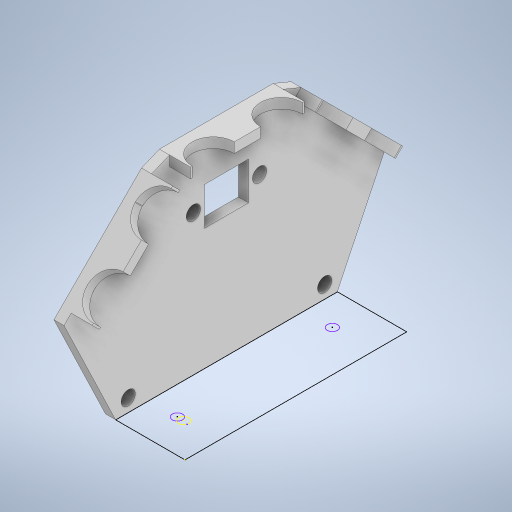
# Autodesk Inventor part: Top front deck
Saved by Autodesk Inventor 2024 (Build 280153000, 153)
## iProperties
Created: 2025-05-10
Part Number: Top front deck
Material: Generic
Document SubType Name: Modeling
Designer: arikm
Density: 1 g/cm^3
Appearance: Default
Author: arikm
Autodesk Inventor part; units mm, degrees
ref_plane "YZ Plane" through (0, 0, 0) normal (1, 0, 0) x (0, 1, 0)
ref_plane "XZ Plane" through (0, 0, 0) normal (0, 1, 0) x (-1, 0, 0)
ref_plane "XY Plane" through (0, 0, 0) normal (0, 0, 1) x (1, 0, 0)
sketch "Sketch1" plane through (0, 0, 0) normal (0, 1, 0) x (-1, 0, 0)
  line L0 (0, 0) -> (27.4, 0)
  line L1 (27.4, 0) -> (27.4, -87.7)
  line L2 (27.4, -87.7) -> (0, -87.7)
  line L3 (0, -87.7) -> (0, 0)
  line L4 (13.7, 0) -> (13.7, -13.2)
  line L5 (13.7, -87.7) -> (13.7, -74.5)
  circle A0 centre (13.7, -13.2) radius 2
  circle A1 centre (13.7, -74.5) radius 2
  dimension "d0" = 27.4
  dimension "d1" = 87.7
  dimension "d2" = 13.2
  dimension "d4" = 4
  dimension "d6" = 4
  constraints: 12 end point, 2 centre point, 2 coincident, 2 midpoint, 2 parallel, 2 vertical, 1 horizontal, 1 perpendicular
  measures "d0" distance of L1.end L2.end
  measures "d1" distance of L0.end L1.end
  measures "d2" distance of L4.start L4.end
  measures "d4" diameter of A0
  measures "d6" diameter of A1
extrude "Extrusion1" add sketch "Sketch1" along normal blind 10
sketch "Sketch2" plane through (0, 0, 0) normal (0, -1, 0) x (1, 0, 0)
  circle A0 centre (-13.7, -13.2) radius 2 projected
  circle A1 centre (-13.7, -13.2) radius 4.5
  circle A2 centre (-13.7, -74.5) radius 2 projected
  circle A3 centre (-13.7, -74.5) radius 4.5
  point P0 (0, 0)
  dimension "d9" = 9
  dimension "d10" = 9
  constraints: 2 centre point, 2 coincident
  measures "d9" diameter of A1
  measures "d10" diameter of A3
extrude "Extrusion2" cut sketch "Sketch2" against normal blind 3
sketch "Sketch3" plane through (0, 10, 0) normal (0, 1, 0) x (1, 0, 0)
  line L0 (0, 0) -> (0, 87.7) projected
  line L1 (0, 87.7) -> (-27.4, 87.7) projected
  line L2 (0, 0) -> (-27.4, 0)
  line L3 (-27.4, 0) -> (-27.4, 87.7)
  line L4 (-27.4, 87.7) -> (0, 87.7)
  line L5 (0, 87.7) -> (0, 0)
  circle A0 centre (-11.7, 12.5929) radius 0.0901
  circle A1 centre (-13.7, 13.2) radius 2 projected
  constraints: 8 end point, 2 parallel, 1 centre point, 1 horizontal, 1 perpendicular, 1 tangent
sketch "Sketch4" plane through (0, 0, 0) normal (0, -1, 0) x (1, 0, 0)
  line L0 (-27.4, -87.7) -> (-27.4, 0) projected
  line L1 (-27.4, -43.85) -> (0, -43.85)
  line L2 (0, 0) -> (0, -87.7) projected
  circle A0 centre (-13.7, -13.2) radius 2 projected
  line L3 (-13.7, -13.2) -> (-13.7, -26.4)
  line L4 (-13.7, -26.4) -> (0, -26.4)
  line L5 (0, -26.4) -> (0, -43.85)
  line L6 (0, -43.85) -> (-13.7, -43.85)
  line L7 (-13.7, -43.85) -> (-13.7, -26.4)
  line L8 (-13.7, -26.4) -> (-27.4, -26.4)
  line L9 (-27.4, -26.4) -> (-27.4, -43.85)
  line L10 (-27.4, -43.85) -> (-13.7, -43.85)
  line L11 (-13.7, -43.85) -> (-13.7, -26.4)
  circle A1 centre (-13.7, -74.5) radius 2 projected
  line L12 (-13.7, -74.5) -> (-13.7, -61.3)
  line L13 (-13.7, -43.85) -> (-13.7, -61.3)
  line L14 (-13.7, -61.3) -> (0, -61.3)
  line L15 (0, -61.3) -> (0, -43.85)
  line L16 (0, -43.85) -> (-13.7, -43.85)
  line L17 (-13.7, -43.85) -> (-13.7, -61.3)
  line L18 (-13.7, -43.85) -> (-27.4, -43.85)
  line L19 (-27.4, -43.85) -> (-27.4, -61.3)
  line L20 (-27.4, -61.3) -> (-13.7, -61.3)
  line L21 (-13.7, -61.3) -> (-13.7, -43.85)
  line L22 (0, -26.4) -> (-27.4, -26.4)
  line L23 (-27.4, -26.4) -> (-27.4, -35.125)
  line L24 (-27.4, -35.125) -> (0, -35.125)
  line L25 (0, -35.125) -> (0, -26.4)
  line L26 (-27.4, -61.3) -> (0, -61.3)
  line L27 (0, -61.3) -> (0, -52.575)
  line L28 (0, -52.575) -> (-27.4, -52.575)
  line L29 (-27.4, -52.575) -> (-27.4, -61.3)
  dimension "d13" = 13.2
  dimension "d14" = 13.2
  constraints: 56 end point, 12 parallel, 6 horizontal, 6 perpendicular, 4 midpoint, 3 vertical, 2 point on line
  measures "d13" distance of L3.start L3.end
  measures "d14" distance of L12.start L12.end
extrude "Extrusion3" add sketch "Sketch4" along normal blind 60 contours L0 L28 L13 L20 | L13 L28 L2 L14 | L0 L8 L7 L24 | L7 L4 L2 L24
sketch "Sketch5" plane through (0, 0, -87.7) normal (1, 0, 0) x (0, 0, -1)
  line L0 (0, 10) -> (-87.7, 10) projected
  line L1 (-87.7, 10) -> (-87.7, 182)
  line L2 (0, 10) -> (-87.7, 10)
  line L3 (-87.7, 10) -> (-87.7, 182)
  line L4 (-87.7, 182) -> (0, 182)
  line L5 (0, 182) -> (0, 10)
  line L6 (-87.7, 182) -> (0, 182)
  line L7 (0, 182) -> (0, 192)
  line L8 (0, 192) -> (-87.7, 192)
  line L9 (-87.7, 192) -> (-87.7, 182)
  line L10 (-61.3, 0) -> (-61.3, -60) projected
  line L11 (-61.3, -60) -> (-61.3, 192)
  line L12 (-26.4, -60) -> (-35.125, -60) projected
  line L13 (-26.4, -60) -> (-26.4, 192)
  line L14 (-52.575, 0) -> (-52.575, -60) projected
  line L15 (-52.575, -60) -> (-61.3, -60)
  line L16 (-61.3, -60) -> (-61.3, 192)
  line L17 (-61.3, 192) -> (-52.575, 192)
  line L18 (-52.575, 192) -> (-52.575, -60)
  line L19 (-26.4, 182) -> (-35.125, 182)
  line L20 (-35.125, 182) -> (-35.125, 192)
  line L21 (-35.125, 192) -> (-26.4, 192)
  line L22 (-26.4, 192) -> (-26.4, 182)
  line L23 (-61.3, 192) -> (-52.575, 192)
  line L24 (-52.575, 192) -> (-52.575, 252)
  line L25 (-52.575, 252) -> (-61.3, 252)
  line L26 (-61.3, 252) -> (-61.3, 192)
  line L27 (-35.125, 192) -> (-26.4, 192)
  line L28 (-26.4, 192) -> (-26.4, 252)
  line L29 (-26.4, 252) -> (-35.125, 252)
  line L30 (-35.125, 252) -> (-35.125, 192)
  line L31 (-26.4, 10) -> (-35.125, 10)
  line L32 (-35.125, 10) -> (-35.125, 192)
  line L33 (-35.125, 192) -> (-26.4, 192)
  line L34 (-26.4, 192) -> (-26.4, 10)
  point P0 (-87.7, 0)
  point P1 (-52.575, 10)
  point P2 (-52.575, 182)
  point P3 (-35.125, 10)
  point P4 (-26.4, 182)
  point P5 (-61.3, 182)
  point P6 (-61.3, 10)
  dimension "d17" = 172
  dimension "d18" = 10
  dimension "d19" = 8.725
  dimension "d20" = 60
  dimension "d21" = 60
  constraints: 62 end point, 14 parallel, 9 perpendicular, 7 horizontal, 7 point on line, 1 vertical
  measures "d17" distance of L0.end L1.end
  measures "d18" distance of L7.end L6.end
  measures "d19" distance of L20.end L21.end
  measures "d20" distance of L24.end L23.end
  measures "d21" distance of L28.end L27.end
extrude "Extrusion4" add sketch "Sketch5" against normal up to surface (27.4 mm away) contours L0 L32 L4 L13 | L4 L13 L8 L7 | L4 L20 L8 L13 | L0 L11 L4 L18 | L4 L18 L8 L20 | L4 L11 L8 L18 | L4 L9 L8 L11
extrude "Extrusion5" add sketch "Sketch5" against normal up to surface (27.4 mm away) contours L8 L30 L29 L28 | L8 L26 L25 L24
sketch "Sketch6" plane through (0, 0, 0) normal (0, -1, 0) x (1, 0, 0)
  circle A0 centre (-13.7, -13.2) radius 4.5 projected
  circle A1 centre (-13.7, -13.2) radius 2
  circle A2 centre (-13.7, -74.5) radius 2 projected
  circle A3 centre (-13.7, -74.5) radius 2
  point P0 (0, 0)
  dimension "d26" = 4
  constraints: 2 centre point, 2 coincident
  measures "d26" diameter of A3
extrude "Extrusion6" add sketch "Sketch6" against normal through all contours A1 | A2
sketch "Sketch7" plane through (-13.7, 0, -74.5) normal (0, -1, 0) x (1, 0, 0)
  circle A0 centre (0, 61.3) radius 2 projected
  circle A1 centre (0, 61.3) radius 2
  circle A2 centre (0, 0) radius 4.5 projected
  circle A3 centre (0, 0) radius 2
  point P0 (13.7, 74.5)
  constraints: 2 centre point, 2 coincident
extrude "Extrusion7" cut sketch "Sketch7" against normal through all contours A0 | A3
sketch "Sketch8" plane through (-27.4, 192, 0) normal (0, 1, 0) x (1, 0, 0)
  circle A0 centre (13.7, 13.2) radius 2 projected
  circle A1 centre (13.7, 13.2) radius 4.5
  circle A2 centre (13.7, 74.5) radius 4.5 projected
  circle A3 centre (13.7, 74.5) radius 4.5
  point P0 (27.4, 0)
  dimension "d31" = 9
  dimension "d32" = 9
  constraints: 2 centre point, 2 coincident
  measures "d31" diameter of A1
  measures "d32" diameter of A3
extrude "Extrusion8" cut sketch "Sketch8" against normal blind 3
sketch "Sketch9" plane through (0, 0, 0) normal (1, 0, 0) x (0, 0, -1)
  line L0 (26.4, 182) -> (26.4, 10) projected
  line L1 (26.4, 10) -> (61.3, 10)
  line L2 (61.3, 10) -> (61.3, 182)
  line L3 (61.3, 182) -> (26.4, 182)
  line L4 (26.4, 182) -> (26.4, 10)
  point P0 (0, 0)
  constraints: 8 end point, 2 parallel, 1 horizontal, 1 perpendicular
extrude "Extrusion9" cut sketch "Sketch9" against normal through all
sketch "Sketch10" plane through (0, 0, 0) normal (1, 0, 0) x (0, 0, -1)
  line L0 (-41.6694, 140.0326) -> (109.1096, 140.0326)
  line L1 (109.1096, 140.0326) -> (109.1096, 292.3119)
  line L2 (109.1096, 292.3119) -> (-41.6694, 292.3119)
  line L3 (-41.6694, 292.3119) -> (-41.6694, 140.0326)
  point P0 (0, 0)
  constraints: 8 end point, 2 parallel, 1 horizontal, 1 perpendicular
extrude "Extrusion10" cut sketch "Sketch10" against normal blind 30
sketch "Sketch11" plane through (0, 10, 0) normal (0, 1, 0) x (1, 0, 0)
  line L0 (0, 61.3) -> (0, 87.7) projected
  line L1 (-27.4, 0) -> (0, 0) projected
  line L2 (0, 87.7) -> (-27.4, 87.7)
  line L3 (-27.4, 87.7) -> (-27.4, 0)
  line L4 (-27.4, 0) -> (0, 0)
  line L5 (0, 0) -> (0, 87.7)
  constraints: 8 end point, 2 parallel, 1 horizontal, 1 perpendicular
extrude "Extrusion11" add sketch "Sketch11" against normal up to surface (10 mm away)
sketch "Sketch12" plane through (0, 10, 0) normal (0, 1, 0) x (1, 0, 0)
  line L0 (0, 61.3) -> (0, 87.7) projected
  line L1 (-27.4, 0) -> (0, 0) projected
  line L2 (0, 87.7) -> (-27.4, 87.7)
  line L3 (-27.4, 87.7) -> (-27.4, 0)
  line L4 (-27.4, 0) -> (0, 0)
  line L5 (0, 0) -> (0, 87.7)
  line L6 (-27.4, 0) -> (-11.2, 0)
  line L7 (0, 87.7) -> (-27.4, 87.7) projected
  line L8 (-27.4, 87.7) -> (-11.2, 87.7)
  line L9 (-11.2, 87.7) -> (-11.2, 74.5)
  line L10 (-11.2, 0) -> (-11.2, 13.2)
  circle A0 centre (-11.2, 74.5) radius 2
  circle A1 centre (-11.2, 13.2) radius 2
  dimension "d41" = 16.2
  dimension "d42" = 16.2
  dimension "d43" = 13.2
  dimension "d44" = 13.2
  dimension "d45" = 4
  dimension "d46" = 4
  constraints: 16 end point, 2 centre point, 2 coincident, 2 parallel, 2 point on line, 2 vertical, 1 horizontal, 1 perpendicular
  measures "d41" distance of L1.start L6.end
  measures "d42" distance of L2.end L8.end
  measures "d43" distance of L8.end L9.end
  measures "d44" distance of L6.end L10.end
  measures "d45" diameter of A0
  measures "d46" diameter of A1
extrude "Extrusion12" cut sketch "Sketch12" against normal through all contours A0 | A1
sketch "Sketch13" plane through (0, 0, -87.7) normal (1, 0, 0) x (0, 0, -1)
  line L0 (-87.7, 10) -> (0, 10) projected
  line L1 (0, 10) -> (-87.7, 10)
  line L2 (-26.4, 0) -> (-26.4, -60) projected
  line L3 (-35.125, 0) -> (-35.125, -60) projected
  line L4 (-26.4, -60) -> (-35.125, -60)
  line L5 (-35.125, -60) -> (-35.125, 0)
  line L6 (-35.125, 0) -> (-26.4, 0)
  line L7 (-26.4, 0) -> (-26.4, -60)
  line L8 (-52.575, 0) -> (-52.575, -60) projected
  line L9 (-61.3, 0) -> (-61.3, -60) projected
  line L10 (-52.575, -60) -> (-61.3, -60)
  line L11 (-61.3, -60) -> (-61.3, 0)
  line L12 (-61.3, 0) -> (-52.575, 0)
  line L13 (-52.575, 0) -> (-52.575, -60)
  line L14 (0, 0) -> (-87.7, 0)
  line L15 (-87.7, 0) -> (-87.7, 10)
  line L16 (-87.7, 10) -> (0, 10)
  line L17 (0, 10) -> (0, 0)
  line L18 (-26.4, 20) -> (-26.4, 80)
  line L19 (-35.125, 20) -> (-35.125, 80)
  line L20 (-26.4, 80) -> (-35.125, 80)
  line L21 (-61.3, 20) -> (-61.3, 80)
  line L22 (-52.575, 80) -> (-61.3, 80)
  line L23 (-52.575, 20) -> (-52.575, 80)
  line L24 (0, 20) -> (-87.7, 20)
  line L25 (-87.7, 20) -> (-87.7, 10)
  line L26 (0, 10) -> (0, 20)
  constraints: 44 end point, 12 symmetric about line, 7 equal length, 3 horizontal, 3 perpendicular, 1 point on line
extrude "Extrusion13" add sketch "Sketch13" against normal up to surface (27.4 mm away) contours L25 L24 L26 L0 | L21 L22 L23 L24 | L24 L19 L20 L18
sketch "Sketch14" plane through (-27.4, 0, -26.4) normal (-1, 0, 0) x (0, 0, 1)
  line L0 (26.4, 0) -> (26.4, 20) projected
  line L1 (26.4, 10) -> (-64.4539, 10)
  line L2 (-64.4539, 10) -> (-64.4539, -69.7314)
  line L3 (-64.4539, -69.7314) -> (26.4, -69.7314)
  line L4 (26.4, -69.7314) -> (26.4, 10)
  constraints: 8 end point, 2 parallel, 1 horizontal, 1 midpoint, 1 perpendicular
extrude "Extrusion14" cut sketch "Sketch14" against normal blind 30
sketch "Sketch15" plane through (0, 20, -61.3) normal (0, 1, 0) x (1, 0, 0)
  line L0 (0, 26.4) -> (0, 0) projected
  line L1 (0, 26.4) -> (0, 13.2)
  line L2 (0, 13.2) -> (-16.2, 13.2)
  line L3 (0, -61.3) -> (0, -48.1)
  line L4 (0, -34.9) -> (0, -61.3) projected
  line L5 (0, -48.1) -> (-16.2, -48.1)
  circle A0 centre (-16.2, 13.2) radius 2
  circle A1 centre (-16.2, -48.1) radius 2
  dimension "d53" = 13.2
  dimension "d54" = 16.2
  dimension "d55" = 13.2
  dimension "d56" = 16.2
  dimension "d57" = 4
  dimension "d58" = 4
  constraints: 8 end point, 2 centre point, 2 coincident, 2 midpoint, 1 horizontal, 1 perpendicular
  measures "d53" distance of L0.start L1.end
  measures "d54" distance of L1.end L2.end
  measures "d55" distance of L3.start L3.end
  measures "d56" distance of L3.end L5.end
  measures "d57" diameter of A0
  measures "d58" diameter of A1
extrude "Extrusion15" cut sketch "Sketch15" against normal blind 30
sketch "Sketch17" plane through (0, 20, -61.3) normal (1, 0, 0) x (0, 0, -1)
  line L0 (-61.3, -10) -> (-61.3, 0) projected
  line L1 (-61.3, -10) -> (-61.3, 179.5615)
  line L2 (-26.175, 60) -> (-34.9, 60) projected
  line L3 (0, 60) -> (-8.725, 60) projected
  line L4 (-26.175, 60) -> (-8.725, 60)
  line L5 (-17.45, 60) -> (-39.95, 60)
  line L6 (-17.45, 60) -> (5.05, 60)
  line L7 (0, 0) -> (0, 60) projected
  line L8 (-34.9, 60) -> (-34.9, 0) projected
  line L9 (0, 60) -> (-34.9, 60)
  line L10 (-34.9, 60) -> (-34.9, 53)
  line L11 (-34.9, 53) -> (0, 53)
  line L12 (0, 53) -> (0, 60)
  line L13 (5.05, 60) -> (-12.9933, 60)
  line L14 (-12.9933, 60) -> (-12.9933, 53)
  line L15 (-12.9933, 53) -> (5.05, 53)
  line L16 (5.05, 53) -> (5.05, 60)
  line L17 (-39.95, 60) -> (-34.9, 60)
  line L18 (-34.9, 60) -> (-34.9, 53)
  line L19 (-34.9, 53) -> (-39.95, 53)
  line L20 (-39.95, 53) -> (-39.95, 60)
  point P0 (-61.3, -20)
  dimension "d61" = 22.5
  dimension "d62" = 22.5
  dimension "d63" = 7
  constraints: 32 end point, 6 parallel, 4 horizontal, 4 point on line, 3 perpendicular, 1 midpoint, 1 vertical
  measures "d61" distance of L5.start L5.end
  measures "d62" distance of L5.start L6.end
  measures "d63" distance of L10.end L9.end
extrude "Extrusion16" add sketch "Sketch17" against normal up to surface (27.4 mm away) contours L4 L14 L11 L8 L2 | L4 L3 L7 L11 L14
extrude "Extrusion17" add sketch "Sketch17" against normal up to surface (27.4 mm away) contours L8 L19 L20 L5 | L7 L6 L16 L15
sketch "Sketch18" plane through (-27.4, 10, -87.7) normal (-1, 0, 0) x (0, 0, 1)
  line L0 (21.35, 70) -> (66.35, 70) projected
  line L1 (66.35, 70) -> (98.1698, 38.1802)
  line L2 (66.35, 70) -> (111.35, 70) construction
  line L3 (21.35, 70) -> (-10.4698, 38.1802)
  line L4 (21.35, 70) -> (66.35, 70) construction
  line L5 (21.35, 70) -> (26.2997, 65.0503)
  line L6 (26.2997, 65.0503) -> (-5.5201, 33.2304)
  line L7 (-10.4698, 38.1802) -> (-5.5201, 33.2304)
  line L8 (43.85, 70) -> (43.85, 34.6614)
  line L9 (66.35, 70) -> (98.1698, 38.1802)
  line L10 (66.35, 70) -> (61.4003, 65.0503)
  line L11 (61.4003, 65.0503) -> (93.2201, 33.2304)
  line L12 (98.1698, 38.1802) -> (93.2201, 33.2304)
  line L13 (21.35, 63) -> (21.35, 70) projected
  line L14 (21.35, 70) -> (21.35, 63)
  line L15 (21.35, 63) -> (24.2495, 63)
  line L16 (66.35, 70) -> (66.35, 63) projected
  line L17 (66.35, 70) -> (66.35, 63)
  line L18 (66.35, 63) -> (63.4505, 63)
  point P0 (87.7, -10)
  dimension "d68" = 45
  dimension "d69" = 45
  dimension "d70" = 45
  dimension "d71" = 135
  dimension "d72" = 7
  dimension "d73" = 45
  constraints: 32 end point, 4 perpendicular, 2 equal length, 2 horizontal, 2 point on line, 2 symmetric about line, 2 vertical, 1 midpoint
  measures "d68" distance of L0.end L1.end
  measures "d69" angle of L1 L2
  measures "d70" distance of L0.start L3.end
  measures "d71" angle of L3 L4
  measures "d72" distance of L0.start L5.end
  measures "d73" distance of L5.end L6.end
extrude "Extrusion18" add sketch "Sketch18" against normal up to surface (27.4 mm away) contours L1 L12 L11 L18 L16 | L13 L15 L6 L7 L3
sketch "Sketch20" plane through (0, 10, -87.7) normal (0, -1, 0) x (1, 0, 0)
  circle A0 centre (-16.2, 13.2) radius 2 projected
  circle A1 centre (-16.2, 13.2) radius 2
  circle A2 centre (-16.2, 74.5) radius 2 projected
  circle A3 centre (-16.2, 74.5) radius 2
  point P0 (0, 87.7)
  constraints: 2 centre point, 2 coincident
extrude "Extrusion19" add sketch "Sketch20" against normal through all
extrude "Extrusion20" cut sketch "Sketch20" against normal through all
sketch "Sketch21" plane through (0, 20, 0) normal (0, 1, 0) x (1, 0, 0)
  circle A0 centre (-16.2, 13.2) radius 2 projected
  circle A1 centre (-16.2, 13.2) radius 5
  circle A2 centre (-16.2, 74.5) radius 2 projected
  circle A3 centre (-16.2, 74.5) radius 5
  point P0 (0, 0)
  dimension "d80" = 10
  dimension "d81" = 10
  constraints: 2 centre point, 2 coincident
  measures "d80" diameter of A1
  measures "d81" diameter of A3
extrude "Extrusion21" add sketch "Sketch21" along normal blind 80 contours A0 | A1 | A3
sketch "Sketch22" plane through (-16.2, 100, -13.2) normal (0, 1, 0) x (1, 0, 0)
  line L0 (-14.7944, -28.3502) -> (23.9654, -28.3502)
  line L1 (23.9654, -28.3502) -> (23.9654, 88.2133)
  line L2 (23.9654, 88.2133) -> (-14.7944, 88.2133)
  line L3 (-14.7944, 88.2133) -> (-14.7944, -28.3502)
  circle A0 centre (0, 0) radius 5 projected
  circle A1 centre (0, 0) radius 5
  circle A2 centre (0, 61.3) radius 2 projected
  circle A3 centre (0, 61.3) radius 5
  point P0 (16.2, -13.2)
  constraints: 8 end point, 2 centre point, 2 coincident, 2 parallel, 1 horizontal, 1 perpendicular
extrude "Extrusion22" cut sketch "Sketch22" against normal blind 80 contours A0 | A3
sketch "Sketch24" plane through (-27.4, 80, -21.35) normal (0, 0.7071068, 0.7071068) x (1, 0, 0)
  line L0 (0, -45) -> (27.4, -45) projected
  line L1 (27.4, 0) -> (0, 0) projected
  line L2 (27.4, -45) -> (0, -45)
  line L3 (0, -45) -> (0, 0)
  line L4 (0, 0) -> (27.4, 0)
  line L5 (27.4, 0) -> (27.4, -45)
  line L6 (0, 0) -> (0, -45)
  line L7 (0, -2.5809) -> (0, -64.5942) projected
  line L8 (0, -22.5) -> (0, -27.5)
  line L9 (0, -27.5) -> (0, -17.5)
  line L10 (0, -27.5) -> (3, -27.5)
  line L11 (3, -27.5) -> (3, -17.5)
  line L12 (3, -17.5) -> (0, -17.5)
  line L13 (0, -17.5) -> (0, -27.5)
  line L14 (0, -17.5) -> (3, -17.5)
  line L15 (3, -17.5) -> (3, -27.5)
  line L16 (3, -27.5) -> (0, -27.5)
  line L17 (0, -27.5) -> (0, -17.5)
  point P0 (27.4, -71.6653)
  dimension "d86" = 5
  dimension "d87" = 10
  dimension "d88" = 3
  constraints: 30 end point, 7 equal length, 3 horizontal, 3 perpendicular, 3 point on line
  measures "d86" distance of L8.start L8.end
  measures "d87" distance of L8.end L9.end
  measures "d88" distance of L12.end L11.end
extrude "Extrusion23" cut sketch "Sketch24" against normal up to surface (7 mm away) contours L3 L12 L11 L10
sketch "Sketch25" plane through (0, 80, -21.35) normal (0, 1, 0) x (1, 0, 0)
  line L0 (-27.4, 13.775) -> (-27.4, 31.225) projected
  line L1 (-27.4, 22.5) -> (-24.4, 22.5)
  line L2 (-24.4, 22.5) -> (-24.4, 17.5)
  line L3 (-24.4, 17.5) -> (-27.4, 17.5)
  line L4 (-27.4, 17.5) -> (-27.4, 22.5)
  line L5 (-27.4, 17.5) -> (-24.4, 17.5)
  line L6 (-24.4, 17.5) -> (-24.4, 27.5)
  line L7 (-24.4, 27.5) -> (-27.4, 27.5)
  line L8 (-27.4, 27.5) -> (-27.4, 17.5)
  point P0 (0, -21.35)
  point P1 (-24.4, 22.5)
  point P2 (-27.4, 27.5)
  dimension "d91" = 3
  dimension "d92" = 5
  dimension "d93" = 10
  constraints: 16 end point, 4 parallel, 2 horizontal, 2 perpendicular, 1 midpoint, 1 point on line
  measures "d91" distance of L2.end L3.end
  measures "d92" distance of L1.end L2.end
  measures "d93" distance of L6.end L5.end
extrude "Extrusion24" cut sketch "Sketch25" against normal blind 10
sketch "Sketch26" plane through (0, 48.1802, -98.1698) normal (0, 0.7071068, -0.7071068) x (-1, 0, 0)
  line L0 (0, 45) -> (27.4, 45) projected
  line L1 (27.4, 45) -> (27.4, 0)
  line L2 (27.4, -19.5942) -> (27.4, 42.4191) projected
  line L3 (0, 42.4191) -> (0, -19.5942) projected
  line L4 (27.4, 45) -> (0, 45)
  line L5 (0, 45) -> (0, 0)
  line L6 (0, 0) -> (27.4, 0)
  line L7 (27.4, 0) -> (27.4, 45)
  line L8 (27.4, 45) -> (27.4, 27.5)
  line L9 (27.4, 24.653) -> (27.4, 62.1297) projected
  line L10 (27.4, 27.5) -> (24.4, 27.5)
  line L11 (24.4, 27.5) -> (24.4, 17.5)
  line L12 (24.4, 17.5) -> (27.4, 17.5)
  line L13 (27.4, 17.5) -> (27.4, 27.5)
  point P0 (0, 35.348)
  dimension "d96" = 45
  dimension "d97" = 17.5
  dimension "d98" = 3
  dimension "d99" = 10
  constraints: 20 end point, 4 parallel, 3 point on line, 2 horizontal, 2 perpendicular
  measures "d96" distance of L0.end L1.end
  measures "d97" distance of L0.end L8.end
  measures "d98" distance of L12.end L11.end
  measures "d99" distance of L11.end L10.end
extrude "Extrusion25" cut sketch "Sketch26" against normal blind 10 contours L1 L12 L11 L10
sketch "Sketch27" plane through (-27.4, 48.1802, 10.4698) normal (0, 0.7071068, 0.7071068) x (1, 0, 0)
  line L0 (0, 0) -> (27.4, 0) projected
  line L1 (27.4, 45) -> (0, 45) projected
  line L2 (27.4, 0) -> (20.4, 0)
  line L3 (20.4, 0) -> (20.4, 45)
  line L4 (20.4, 45) -> (27.4, 45)
  line L5 (27.4, 45) -> (27.4, 0)
  point P0 (27.4, -26.6653)
  dimension "d102" = 7
  constraints: 8 end point, 2 parallel, 1 horizontal, 1 perpendicular, 1 point on line
  measures "d102" distance of L3.end L4.end
extrude "Extrusion26" add sketch "Sketch27" along normal blind 10
sketch "Sketch28" plane through (-27.4, 80, -66.35) normal (0, 1, 0) x (1, 0, 0)
  line L0 (27.4, -45) -> (20.4, -45) projected
  line L1 (27.4, 0) -> (27.4, -45) projected
  line L2 (20.4, -45) -> (27.4, -45)
  line L3 (27.4, -45) -> (27.4, 0)
  line L4 (27.4, 0) -> (20.4, 0)
  line L5 (20.4, 0) -> (20.4, -45)
  point P0 (27.4, -66.35)
  constraints: 8 end point, 2 parallel, 1 horizontal, 1 perpendicular
extrude "Extrusion27" add sketch "Sketch28" along normal blind 10
sketch "Sketch29" plane through (0, 48.1802, -98.1698) normal (0, 0.7071068, -0.7071068) x (-1, 0, 0)
  line L0 (0, 45) -> (7, 45) projected
  line L1 (7, 45) -> (0, 45)
  line L2 (0, 45) -> (0, 0)
  line L3 (0, 0) -> (7, 0)
  line L4 (7, 0) -> (7, 45)
  point P0 (0, 35.348)
  constraints: 8 end point, 2 parallel, 1 horizontal, 1 perpendicular
extrude "Extrusion28" add sketch "Sketch29" along normal blind 10
sketch "Sketch30" plane through (-7, 55.2513, 17.5409) normal (-1, 0, 0) x (0, 0.7071068, 0.7071068)
  line L0 (-10, 45) -> (0, 45) projected
  line L1 (-5, 45) -> (-6.4645, 48.5355)
  line L2 (-10, 45) -> (-2.9289, 52.0711) projected
  line L3 (0, 45) -> (-2.9289, 52.0711)
  line L4 (-2.9289, 52.0711) -> (-34.7487, 83.8909) projected
  line L5 (-34.7487, 83.8909) -> (-41.8198, 76.8198)
  line L6 (-41.8198, 76.8198) -> (-41.8198, 86.8198)
  line L7 (-41.8198, 86.8198) -> (-34.7487, 83.8909)
  point P0 (-51.4718, -26.6653)
  constraints: 10 end point, 2 midpoint, 1 perpendicular, 1 vertical
extrude "Extrusion29" add sketch "Sketch30" against normal up to surface (7 mm away)
sketch "Sketch31" plane through (-7, 80, -66.35) normal (-1, 0, 0) x (0, 0, 1)
  line L0 (52.0711, 7.0711) -> (83.8909, -24.7487) projected
  line L1 (57.3744, -12.3744) -> (45, 0) projected
  line L2 (52.0711, 7.0711) -> (45, 0)
  line L3 (52.0711, 7.0711) -> (45, 10) projected
  line L4 (45, 0) -> (45, 10)
  line L5 (45, 10) -> (52.0711, 7.0711)
  line L6 (0, 10) -> (-7.0711, 7.0711) projected
  line L7 (-7.0711, 7.0711) -> (0, 10)
  line L8 (0, 0) -> (-12.3744, -12.3744) projected
  line L9 (0, 10) -> (0, 0)
  line L10 (0, 0) -> (-7.0711, 7.0711)
  point P0 (66.35, -80)
  constraints: 12 end point, 2 collinear, 2 perpendicular, 2 vertical
extrude "Extrusion30" add sketch "Sketch31" along normal up to surface (20.4 mm away)
sketch "Sketch32" plane through (-27.4, 43.2304, 5.5201) normal (0, -0.7071068, 0.7071068) x (1, 0, 0)
  line L0 (27.4, 0) -> (0, 0) projected
  line L1 (27.4, 17) -> (20.4, 17) projected
  line L2 (0, 0) -> (27.4, 0)
  line L3 (27.4, 0) -> (27.4, 17)
  line L4 (27.4, 17) -> (0, 17)
  line L5 (0, 17) -> (0, 0)
  point P0 (27.4, -34.4718)
  point P1 (20.4, 17)
  constraints: 8 end point, 2 parallel, 1 horizontal, 1 perpendicular
extrude "Extrusion31" add sketch "Sketch32" along normal blind 4
sketch "Sketch33" plane through (0, 43.2304, -93.2201) normal (0, -0.7071068, -0.7071068) x (-1, 0, 0)
  line L0 (0, 14.0711) -> (0, 17) projected
  line L1 (27.4, 7) -> (27.4, -5.3744) projected
  line L2 (0, 17) -> (27.4, 17)
  line L3 (27.4, 17) -> (27.4, 0)
  line L4 (27.4, 0) -> (0, 0)
  line L5 (0, 0) -> (0, 17)
  point P0 (0, -96.4851)
  point P1 (0, 14.0711)
  dimension "d115" = 17
  constraints: 8 end point, 2 parallel, 1 horizontal, 1 perpendicular, 1 point on line
  measures "d115" distance of L2.end L3.end
extrude "Extrusion32" add sketch "Sketch33" along normal blind 4
sketch "Sketch34" plane through (-27.4, 10, -87.7) normal (-1, 0, 0) x (0, 0, 1)
  line L0 (87.7, 0) -> (87.7, 10) projected
  line L1 (73.4211, 77.0711) -> (108.0693, 42.4228) projected
  line L2 (87.7, 0) -> (108.0693, 42.4228)
  line L3 (0, 0) -> (0, 10) projected
  line L4 (-17.5409, 45.2513) -> (-20.3693, 42.4228) projected
  line L5 (0, 0) -> (-20.3693, 42.4228)
  line L6 (108.0693, 42.4228) -> (73.4211, 77.0711)
  line L7 (73.4211, 77.0711) -> (66.35, 80) projected
  line L8 (73.4211, 77.0711) -> (66.35, 80)
  line L9 (66.35, 80) -> (21.35, 80) projected
  line L10 (66.35, 80) -> (21.35, 80)
  line L11 (21.35, 80) -> (14.2789, 77.0711) projected
  line L12 (21.35, 80) -> (14.2789, 77.0711)
  line L13 (14.2789, 77.0711) -> (-20.3693, 42.4228)
  line L14 (108.0693, 42.4228) -> (96.0485, 30.402)
  line L15 (61.3, 10) -> (87.7, 10) projected
  line L16 (108.0693, 42.4228) -> (153.9221, 42.4228) construction
  line L17 (63.4505, 63) -> (96.0485, 30.402) projected
  line L18 (65.0399, 10) -> (75.6465, 10)
  line L19 (-20.3693, 42.4228) -> (12.0535, 10)
  line L20 (-20.3693, 42.4228) -> (25.4835, 42.4228) construction
  line L21 (-8.3485, 30.402) -> (-3.0452, 35.7053)
  line L22 (-3.0452, 35.7053) -> (22.6601, 10)
  line L23 (22.6601, 10) -> (12.0535, 10)
  line L24 (96.0485, 30.402) -> (87.7, 10)
  line L25 (87.7, 10) -> (80.2, 10)
  line L26 (80.2, 10) -> (93.788, 43.2062)
  line L27 (96.0485, 30.402) -> (90.7263, 35.7242)
  line L28 (35.125, 10) -> (52.575, 10) projected
  line L29 (43.85, 10) -> (43.85, 63)
  line L30 (48.85, 63) -> (38.85, 63) projected
  line L31 (-8.3485, 30.402) -> (0, 10)
  line L32 (0, 10) -> (7.5, 10)
  line L33 (7.5, 10) -> (-6.088, 43.2062)
  line L34 (-8.3485, 30.402) -> (-3.0263, 35.7242)
  line L35 (94.5362, 31.9143) -> (85.1191, 10)
  line L36 (96.0485, 30.402) -> (94.5362, 31.9143)
  line L37 (80.8457, 45.6048) -> (96.0485, 30.402) projected
  line L38 (26.4, 10) -> (0, 10)
  line L39 (-8.3485, 30.402) -> (0, 10)
  line L40 (-8.3485, 30.402) -> (-3.0263, 35.7242)
  line L41 (-6.8362, 31.9143) -> (2.5809, 10)
  point P0 (87.7, -10)
  point P1 (2.5809, 10)
  point P2 (-4.5571, 26.6106)
  point P3 (94.5362, 31.9143)
  point P4 (85.1191, 10)
  dimension "d121" = 45
  dimension "d122" = 7.5
  dimension "d123" = 7.5
  dimension "d124" = 1
  constraints: 60 end point, 11 point on line, 10 symmetric about line, 4 collinear, 4 horizontal, 3 perpendicular, 2 midpoint, 1 equal length, 1 parallel
  measures "d121" angle of L19 L20
  measures "d122" distance of L21.start L21.end
  measures "d123" distance of L0.end L25.end
  measures "d124" angle of L24 L35
extrude "Extrusion33" add sketch "Sketch34" against normal blind 10 contours L0 L24 L14 L2 | L15 L35 L17 L24 | L5 L19 L31 L3 | L31 L19 L41 L32
sketch "Sketch35" plane through (-27.4, 20, -52.575) normal (-1, 0, 0) x (0, 0, 1)
  line L0 (52.575, 0) -> (52.575, -10) projected
  line L1 (26.175, 0) -> (49.9941, 0) projected
  line L2 (52.575, -10) -> (42.575, -10)
  line L3 (42.575, -10) -> (42.575, 0)
  line L4 (42.575, 0) -> (52.575, 0)
  line L5 (52.575, 0) -> (52.575, -10)
  line L6 (72.9443, 32.4228) -> (52.575, -10) projected
  line L7 (52.575, -10) -> (42.575, 0)
  circle A0 centre (47.575, -5) radius 2.8
  line L8 (52.575, -10) -> (-35.125, -10) projected
  line L9 (8.725, -10) -> (8.725, 0)
  line L10 (0, 0) -> (17.45, 0) projected
  circle A1 centre (-30.125, -5) radius 2.8
  line L11 (17.45, 0) -> (17.45, 53) projected
  line L12 (26.175, 53) -> (26.175, 0) projected
  line L13 (17.45, 53) -> (26.175, 53)
  line L14 (26.175, 53) -> (26.175, 38)
  line L15 (26.175, 38) -> (17.45, 38)
  line L16 (17.45, 38) -> (17.45, 53)
  line L17 (-8.725, 53) -> (-10.8755, 53) projected
  line L18 (26.175, 38) -> (-8.725, 38)
  line L19 (-8.725, 38) -> (-8.725, 53)
  line L20 (-8.725, 53) -> (26.175, 53)
  line L21 (26.175, 53) -> (26.175, 38)
  line L22 (-8.725, 38) -> (0, 38)
  line L23 (0, 38) -> (0, 53)
  line L24 (0, 53) -> (-8.725, 53)
  line L25 (-8.725, 53) -> (-8.725, 38)
  line L26 (26.175, 38) -> (17.45, 53)
  line L27 (3.725, 53) -> (0, 53) projected
  line L28 (0, 53) -> (-8.725, 38)
  circle A2 centre (21.8125, 45.5) radius 2.8
  circle A3 centre (-4.3625, 45.5) radius 2.8
  line L29 (31.225, 60) -> (31.225, 70) projected
  line L30 (38.2961, 67.0711) -> (31.225, 70) projected
  line L31 (31.225, 70) -> (38.2961, 67.0711)
  line L32 (38.2961, 67.0711) -> (72.9443, 32.4228)
  line L33 (72.9443, 32.4228) -> (52.575, -10)
  line L34 (52.575, -10) -> (-35.125, -10)
  line L35 (-35.125, -10) -> (-55.4943, 32.4228) projected
  line L36 (-35.125, -10) -> (-55.4943, 32.4228)
  line L37 (-55.4943, 32.4228) -> (-20.8461, 67.0711)
  line L38 (-20.8461, 67.0711) -> (-13.775, 70)
  line L39 (-13.775, 70) -> (31.225, 70)
  point P0 (52.575, -20)
  point P1 (0, 38)
  dimension "d127" = 10
  dimension "d128" = 5.6
  dimension "d129" = 15
  dimension "d130" = 5.6
  dimension "d131" = 5.6
  constraints: 56 end point, 9 parallel, 5 midpoint, 5 perpendicular, 4 centre point, 4 collinear, 4 horizontal, 3 point on line, 1 symmetric about line, 1 other
  measures "d127" distance of L3.end L4.end
  measures "d128" diameter of A0
  measures "d129" distance of L13.end L14.end
  measures "d130" diameter of A2
  measures "d131" diameter of A3
extrude "Extrusion34" add sketch "Sketch35" along normal blind 4 contours L4 L1 L12 L13 L20 L19 L18 L11 L10 L9 L8 L35 L37 L38 L39 L30 L32 L6 L0 | L0 L7 A0 L1 L4 | L2 L3 L7 A0 | L8 L9 L10 L11 L15 L12 L1 L3 | L26 A2 L13 L12 | L15 L11 L26 A2 | L18 L28 A3 L23 | L19 L20 L28 A3
sketch "Sketch36" plane through (0, 10, -87.7) normal (0, -1, 0) x (1, 0, 0)
  line L0 (0, 0) -> (-17.4, 0) projected
  line L1 (-17.4, 0) -> (-17.4, -25)
  line L2 (-17.4, -8.3485) -> (-17.4, -20.3693) projected
  line L3 (-17.4, -25) -> (-17.4, 119.772)
  line L4 (-17.4, 119.772) -> (7.6601, 119.772)
  line L5 (7.6601, 119.772) -> (7.6601, -47.6838)
  line L6 (7.6601, -47.6838) -> (-17.4, -47.6838)
  line L7 (-17.4, -47.6838) -> (-17.4, 119.772)
  line L8 (-31.4, 87.7) -> (-17.4, 87.7) projected
  line L9 (-31.4, 87.7) -> (-27.4, 87.7)
  line L10 (-27.4, 87.7) -> (4.1783, 87.7)
  line L11 (4.1783, 87.7) -> (4.1783, -30.9605)
  line L12 (4.1783, -30.9605) -> (-27.4, -30.9605)
  line L13 (-27.4, -30.9605) -> (-27.4, 87.7)
  line L14 (-27.4, -30.9605) -> (13.0906, -30.9605)
  line L15 (13.0906, -30.9605) -> (13.0906, 140.084)
  line L16 (13.0906, 140.084) -> (-27.4, 140.084)
  line L17 (-27.4, 140.084) -> (-27.4, -30.9605)
  point P0 (0, 87.7)
  point P1 (-17.4, -30.9605)
  point P2 (7.6601, -30.9605)
  dimension "d134" = 25
  dimension "d135" = 4
  constraints: 30 end point, 6 parallel, 3 horizontal, 3 perpendicular, 2 point on line, 1 collinear
  measures "d134" distance of L0.end L1.end
  measures "d135" distance of L8.start L9.end
extrude "Extrusion35" cut sketch "Sketch36" against normal through all
sketch "Sketch37" plane through (-27.4, 90, -21.35) normal (0, 1, 0) x (1, 0, 0)
  line L0 (-4, 0) -> (-4, 45) projected
  line L1 (-4, 22.5) -> (-4, 0)
  line L2 (-4, 0) -> (-4, 45)
  line L3 (0, 66.35) -> (0, -21.35) projected
  line L4 (-4, 0) -> (0, 0)
  line L5 (0, 0) -> (0, 45)
  line L6 (0, 45) -> (-4, 45)
  line L7 (-4, 45) -> (-4, 0)
  line L8 (0, 45) -> (27.4, 45)
  line L9 (27.4, 45) -> (27.4, 0)
  line L10 (27.4, 0) -> (0, 0)
  line L11 (0, 0) -> (0, 45)
  line L12 (-4, 0) -> (8.3, 0)
  line L13 (0, 0) -> (0, 9)
  line L14 (8.3, 0) -> (8.3, 9)
  line L15 (8.3, 9) -> (-4, 9)
  line L16 (-4, 9) -> (-4, 0)
  line L17 (-4, 0) -> (8.3, 0)
  line L18 (8.3, 0) -> (8.3, 9)
  circle A0 centre (8.3, 9) radius 8.3
  line L19 (8.3, 9) -> (8.3, 45)
  line L20 (8.3, 45) -> (8.3, 36)
  circle A1 centre (8.3, 36) radius 8.3
  line L21 (8.3, 0) -> (0, 0)
  line L22 (0, 0) -> (0, 45)
  line L23 (0, 45) -> (8.3, 45)
  line L24 (8.3, 45) -> (8.3, 0)
  point P0 (27.4, -21.35)
  point P1 (8.3, 0.7)
  point P2 (8.3, 17.3)
  point P3 (8.3, 27.7)
  point P4 (8.3, 44.3)
  dimension "d138" = 22.5
  dimension "d139" = 12.3
  dimension "d140" = 9
  dimension "d141" = 9
  dimension "d142" = 16.6
  dimension "d143" = 9
  dimension "d144" = 16.6
  constraints: 46 end point, 8 parallel, 5 perpendicular, 5 point on line, 4 horizontal, 2 centre point, 2 coincident, 2 collinear, 1 midpoint, 1 vertical
  measures "d138" distance of L1.start L0.start
  measures "d139" distance of L0.start L12.end
  measures "d140" distance of L10.end L13.end
  measures "d141" distance of L12.end L14.end
  measures "d142" diameter of A0
  measures "d143" distance of L19.end L20.end
  measures "d144" diameter of A1
extrude "Extrusion36" add sketch "Sketch37" against normal blind 4 contours L0 L15 L3 L4 | L0 L6 L3 L15 | L3 A0 L14 L10 | L3 A1 L19 A0 | L3 L8 L19 A1
sketch "Sketch39" plane through (-27.4, 55.2513, 17.5409) normal (0, 0.7071068, 0.7071068) x (1, 0, 0)
  line L0 (0, 45) -> (-4, 45) projected
  line L1 (-4, 45) -> (27.4, 45)
  line L2 (27.4, 45) -> (27.4, 0)
  line L3 (27.4, 0) -> (-4, 0)
  line L4 (-4, 0) -> (-4, 45)
  line L5 (0, 42.4191) -> (0, -19.5942) projected
  line L6 (0, 0) -> (0, 9)
  line L7 (0, 9) -> (16.6, 9)
  circle A0 centre (8.3, 9) radius 8.3
  line L8 (0, 45) -> (0, 36)
  line L9 (0, 36) -> (16.5978, 35.7307)
  circle A1 centre (8.2989, 35.8654) radius 8.3
  line L10 (8.3, 9) -> (8.3, 0)
  line L11 (8.3, 0) -> (8.3, 45)
  point P0 (27.4, -26.6653)
  point P1 (8.3, 44.1654)
  point P2 (0, 42.4191)
  point P3 (8.3, 17.3)
  point P4 (8.3, 27.5654)
  point P5 (0, 35.7307)
  point P6 (8.3, 0.7)
  dimension "d161" = 45
  dimension "d162" = 9
  dimension "d163" = 16.6
  dimension "d164" = 9
  dimension "d165" = 16.6
  constraints: 20 end point, 6 point on line, 4 perpendicular, 2 midpoint, 2 parallel, 1 horizontal, 6 other
  measures "d161" distance of L1.end L2.end
  measures "d162" distance of L6.start L6.end
  measures "d163" distance of L6.end L7.end
  measures "d164" distance of L0.start L8.end
  measures "d165" distance of L8.end L9.end
extrude "Extrusion39" add sketch "Sketch39" against normal blind 4 contours L1 L11 A1 L5 L8 | A1 L11 A0 L5 | L5 A0 L10 L3
sketch "Sketch40" plane through (0, 55.2513, -105.2409) normal (0, 0.7071068, -0.7071068) x (-1, 0, 0)
  line L0 (31.4, 45) -> (31.4, -4) projected
  line L1 (31.4, 45) -> (6.6569, 45)
  line L2 (6.6569, 45) -> (6.6569, 0)
  line L3 (6.6569, 0) -> (31.4, 0)
  line L4 (31.4, 0) -> (31.4, 45)
  line L5 (27.4, 45) -> (27.4, -4) projected
  line L6 (27.4, 45) -> (27.4, 36)
  line L7 (27.4, 36) -> (10.8, 36)
  circle A0 centre (19.1, 36) radius 8.3
  line L8 (27.4, 0) -> (10.8, 0)
  line L9 (10.8, 0) -> (10.8, 9)
  line L10 (19.1, 0) -> (19.1, 9)
  circle A1 centre (19.1, 9) radius 8.3
  line L11 (19.1, 36) -> (19.1, 45)
  line L12 (19.1, 45) -> (19.1, 0)
  point P0 (0, 35.348)
  point P1 (19.1, 27.7)
  point P2 (19.1, 17.3)
  point P3 (27.4, 9)
  point P4 (19.1, 44.3)
  point P5 (19.1, 0.7)
  point P6 (19.1, 0)
  dimension "d168" = 45
  dimension "d169" = 9
  dimension "d170" = 16.6
  dimension "d171" = 16.6
  dimension "d172" = 9
  dimension "d173" = 9
  constraints: 22 end point, 5 point on line, 3 perpendicular, 2 midpoint, 2 parallel, 1 centre point, 1 coincident, 1 horizontal, 1 tangent, 1 vertical, 3 other
  measures "d168" distance of L2.end L1.end
  measures "d169" distance of L5.start L6.end
  measures "d170" distance of L6.end L7.end
  measures "d171" distance of L8.start L8.end
  measures "d172" distance of L8.end L9.end
  measures "d173" distance of L11.start L11.end
extrude "Extrusion40" add sketch "Sketch40" against normal blind 4 contours L5 A0 L11 L1 | L3 L10 A1 L5 | L5 A1 L12 A0
body "Solid1"
